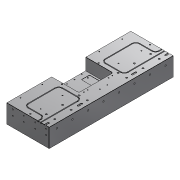
# Autodesk Inventor part: BC-10001
Saved by Autodesk Inventor 2016 (Build 200138000, 138)
## iProperties
Created: 2015-11-16
Part Number: BC-10001
Project: DIPOLO BC-3T- SIRIUS
Cost Center: 1504002005
Material: Aço Carbono AISI 1006
Document SubType Name: Modeling
Designer: reinaldo.basilio
Density: 7.872 g/cm^3
Appearance: Silver
Mass: 270714 g
Surface Area: 10813.1 cm^2
Volume: 34389.5 cm^3
Description: Base de referência de montagem do BC.
RuleStatus: InUse
AfterMaterialChange0: file://_iMaterial
AfterAnyiPropertyChange0: file://_iMaterial
AfterDocNew0: file://_Naming_par
AfterDocNew1: file://_NameStart
AfterDocNew2: file://_NameStart1
AfterDocNew3: file://_Materiais
DocNumber: XXXXX-XXX-XXXX-00-001.ipt
Folder: .
Title: DIPOLO BC-3T- SIRIUS
Author: reinaldo.basilio
Subject: BC-10001
Autodesk Inventor part; units mm, degrees
ref_plane "YZ Plane" through (0, 0, 0) normal (1, 0, 0) x (0, 1, 0)
ref_plane "XZ Plane" through (0, 0, 0) normal (0, 1, 0) x (-1, 0, 0)
ref_plane "XY Plane" through (0, 0, 0) normal (0, 0, 1) x (1, 0, 0)
sketch "Sketch5" plane through (0, 0, 0) normal (0, 0, 1) x (1, 0, 0)
  line L0 (-456.5, 228) -> (456.5, 228)
  line L1 (456.5, 228) -> (456.5, -55)
  line L2 (456.5, -55) -> (-456.5, -55)
  line L3 (-456.5, -55) -> (-456.5, 228)
  point P0 (0, 0)
  point P1 (0, 228)
  dimension "d8" = 913
  dimension "d154" = 55
  dimension "d523" = 283
  constraints: 8 end point, 2 parallel, 1 horizontal, 1 midpoint, 1 perpendicular, 1 vertical alignment
  measures "d8" distance of L0.start L0.end
  measures "d154" distance from line of L2 point (0, 0)
  measures "d523" distance of L0.end L1.end
extrude "Extrusion5" add sketch "Sketch5" along normal blind 137.5
sketch "Sketch7" plane through (0, 0, 137.5) normal (0, 0, 1) x (1, 0, 0)
  line L0 (125, -55) -> (125, 115)
  line L1 (0, 0) -> (0, 57.6278)
  line L2 (-125, -55) -> (-125, 115)
  line L3 (125, 115) -> (-125, 115)
  line L4 (125, -55) -> (-125, -55)
  line L5 (-456.5, 228) -> (-456.5, -55)
  line L6 (456.5, 228) -> (-456.5, 228) projected
  line L7 (-456.5, -55) -> (456.5, -55) projected
  point P0 (0, 115)
  point P1 (0, 28.8139)
  point P2 (0, -55)
  point P3 (0, -55)
  point P4 (0, 228)
  point P5 (0, 228)
  dimension "d76" = 250
  dimension "d77" = 170
  constraints: 12 end point, 6 midpoint, 4 vertical alignment, 2 vertical, 1 collinear, 1 horizontal, 1 symmetric about line
  measures "d76" distance of L0.end L2.end
  measures "d77" distance of L0.start L0.end
extrude "Extrusion7" cut sketch "Sketch7" against normal blind 87.5
sketch "Sketch11" plane through (0, 0, 50) normal (0, 0, 1) x (1, 0, 0)
  line L0 (90, 145) -> (-105, 145)
  line L1 (52.5, -55) -> (-52.5, -55) construction
  line L2 (-52.5, -55) -> (-52.5, 55)
  line L3 (-52.5, 55) -> (52.5, 55) construction
  line L4 (52.5, 55) -> (52.5, -55)
  line L5 (112.5, -45) -> (52.5, -45)
  line L6 (52.5, -45) -> (52.5, 45)
  line L7 (52.5, 45) -> (112.5, 45)
  line L8 (112.5, 45) -> (112.5, -45)
  line L9 (-125, -55) -> (-125, 115)
  line L10 (125, 115) -> (125, -55) projected
  line L11 (-125, -55) -> (-125, 115) projected
  line L12 (-125, 115) -> (125, 115) projected
  line L13 (0, 55) -> (0, -3.7877) construction
  line L14 (-112.5, -45) -> (-52.5, -45)
  line L15 (-52.5, 45) -> (-112.5, 45)
  line L16 (-112.5, 45) -> (-112.5, -45)
  line L17 (-52.5, -45) -> (-52.5, 45)
  line L18 (125, -55) -> (-125, -55) projected
  circle A0 centre (112.5, -45) radius 4
  circle A1 centre (52.5, -45) radius 4
  circle A2 centre (52.5, 45) radius 4
  circle A3 centre (112.5, 45) radius 4
  point P0 (112.5, 0)
  point P1 (52.5, 0)
  point P2 (0, 115)
  dimension "d55" = 110
  dimension "d56" = 105
  dimension "d58" = 60
  dimension "d59" = 90
  dimension "d156" = 72.5
  dimension "d158" = 72.5
  dimension "d160" = 60
  dimension "d225" = 55
  dimension "d310" = 8
  constraints: 30 end point, 5 midpoint, 4 centre point, 4 coincident, 4 symmetric about line, 3 equal radius, 3 parallel, 2 horizontal, 2 horizontal alignment, 2 perpendicular, 1 collinear, 1 vertical, 1 vertical alignment
  measures "d55" distance of L3.end L1.start
  measures "d56" distance of L2.end L3.end
  measures "d58" distance of L6.end L7.end
  measures "d59" distance of L7.end L5.start
  measures "d156" distance between parallel lines of L10 L4
  measures "d158" distance between parallel lines of L11 L2
  measures "d160" distance of L15.start L16.start
  measures "d225" distance from line of point (52.5, 0) L18
  measures "d310" diameter of A0
extrude "Extrusion9" cut sketch "Sketch11" against normal blind 2 contours L14 L16 L15 L2 | L4 A1 L5 | L4 A2 L7 A3 L8 A0 L5 A1 | L4 L7 A2 | A0 L8 L5 | L7 L8 A3 picked at (54.7437, -43.5902) picked at (54.3738, 43.1262) picked at (109.8668, -44.7033) picked at (110.2563, 43.5902)
fillet "Fillet2" radius 4 8 edges at (112.5, 45, 49) (52.5, 45, 49) (-112.5, 45, 49) (-52.5, 45, 49) (-112.5, -45, 49) (52.5, -45, 49) (-52.5, -45, 49) (112.5, -45, 49)
sketch "Sketch12" plane through (0, 0, 50) normal (0, 0, 1) x (1, 0, 0)
  line L0 (-434.5, -55) -> (478.5, -55)
  circle A0 centre (90.5, -35) radius 4.25
  circle A1 centre (90.5, 35) radius 4.25
  circle A2 centre (-90.5, -35) radius 4
  circle A3 centre (-90.5, 35) radius 4
  line L1 (-52.5, 41) -> (-52.5, -41)
  line L2 (52.5, -41) -> (52.5, 41)
  line L3 (125, -55) -> (-125, -55)
  line L4 (52.5, 0) -> (-52.5, 0) construction
  point P0 (0, -55)
  point P1 (0, 0)
  dimension "d64" = 70
  dimension "d65" = 90.5
  dimension "d66" = 8.5
  dimension "d157" = 90.5
  dimension "d270" = 55
  dimension "d271" = 35
  constraints: 10 end point, 4 centre point, 4 midpoint, 3 vertical alignment, 2 horizontal alignment, 1 equal radius, 3 other
  measures "d64" distance of A0.centre A1.centre
  measures "d65" horizontal distance of point (0, 0) A0.centre
  measures "d66" diameter of A0
  measures "d157" horizontal distance of point (0, 0) A3.centre
  measures "d270" distance from line of point (0, 0) L0
  measures "d271" vertical distance of point (0, 0) A0.centre
hole "Hole2" at (90.5, -35, 50) at (90.5, 35, 50) at (-90.5, 35, 50) at (-90.5, -35, 50) direction (0, 0, -1) diameter 8.376 depth 30 tip angle 118 thread size "M10x1.5" class "6H" standard "ISO Metric profile"
fillet "Fillet4" radius 10 2 edges at (125, 115, 93.75) (-125, 115, 93.75)
sketch "Sketch16" plane through (0, 0, 137.5) normal (0, 0, 1) x (1, 0, 0)
  line L0 (125, 105) -> (125, -55) projected
  line L1 (-456.5, -55) -> (-125, -55) projected
  circle A0 centre (0, 0) radius 8.7018
  line L2 (456.2612, -43.3901) -> (126.3743, -52.0283)
  line L3 (126.3743, -52.0283) -> (123.6257, 52.9357)
  line L4 (123.6257, 52.9357) -> (453.5127, 61.5739)
  line L5 (453.5127, 61.5739) -> (456.2612, -43.3901)
  circle A1 centre (440, 72.475) radius 5
  circle A2 centre (440, 72.475) radius 11.251
  line L6 (125, 0.4537) -> (454.8869, 9.0919)
  circle A3 centre (134.9966, 0.7155) radius 5
  line L7 (0, 0) -> (0, -90.9039)
  arc A4 (0, 0) -> (607.3073, 10.7125) centre (0, 17220) ccw construction
  line L8 (0, 0) -> (517.2786, 0) construction
  circle A5 centre (-440, 72.475) radius 11.251
  circle A6 centre (-134.9966, 0.7155) radius 5
  circle A7 centre (-440, 72.475) radius 11.251
  circle A8 centre (-134.9966, 0.7155) radius 5
  line L9 (125, 0.4537) -> (124.2986, 0.4537)
  line L10 (456.5, -55) -> (456.5, 228) projected
  point P0 (0, 0)
  point P1 (-456.5, 228)
  dimension "d95" = 55
  dimension "d100" = 10
  dimension "d117" = 105
  dimension "d119" = 17220
  dimension "d123" = 1.5
  dimension "d144" = 10
  dimension "d147" = 52.5
  dimension "d151" = 283
  dimension "d152" = 330
  dimension "d198" = 16.5
  dimension "d199" = 72.475
  dimension "d200" = 22.5021
  dimension "d201" = 134.9966
  dimension "d202" = 440
  constraints: 16 end point, 9 centre point, 4 parallel, 3 midpoint, 3 point on circle, 3 symmetric about line, 2 coincident, 2 concentric, 2 point on line, 1 horizontal, 1 perpendicular, 1 tangent, 1 vertical, 1 vertical alignment, 3 other
  measures "d95" distance from line of L7.start L1
  measures "d100" diameter of A1
  measures "d117" distance between parallel lines of L4 L2
  measures "d119" radius of A4
  measures "d123" angle of L6 L8
  measures "d144" diameter of A3
  measures "d147" distance between parallel lines of L4 L6
  measures "d151" distance of point (-456.5, 228) L1.start
  measures "d152" distance between parallel lines of L3 L5
  measures "d198" distance from line of L10 A1.centre
  measures "d199" vertical distance of A2.centre L7.start
  measures "d200" diameter of A2
  measures "d201" horizontal distance of L7.start A3.centre
  measures "d202" horizontal distance of L7.start A1.centre
hole "Hole3_ref angular" at (440, 72.475, 137.5) at (-440, 72.475, 137.5) at (134.9966, 0.7155, 137.5) at (-134.9966, 0.7155, 137.5) direction (0, 0, -1) diameter 10 depth 10
sketch "Sketch17" plane through (-456.5, -55, 0) normal (0, -1, 0) x (1, 0, 0)
  line L0 (581.5, 137.5) -> (581.5, 50)
  line L1 (581.5, 50) -> (331.5, 50)
  line L2 (331.5, 50) -> (331.5, 137.5)
  line L3 (0, 137.5) -> (331.5, 137.5)
  line L4 (0, 0) -> (0, 137.5)
  line L5 (913, 0) -> (0, 0)
  line L6 (913, 0) -> (913, 137.5)
  line L7 (581.5, 137.5) -> (913, 137.5)
  point P0 (456.5, 0)
  constraints: 16 end point
extrude "Extrusion11" add sketch "Sketch17" along normal blind 30
sketch "Sketch10" plane through (-456.5, -85, 0) normal (0, -1, 0) x (1, 0, 0)
  circle A0 centre (406.5, 25) radius 5
  circle A1 centre (506.5, 25) radius 5
  line L0 (913, 0) -> (0, 0)
  line L1 (581.5, 50) -> (331.5, 50)
  line L2 (581.5, 137.5) -> (581.5, 50) projected
  line L3 (581.5, 50) -> (331.5, 50) projected
  line L4 (331.5, 50) -> (331.5, 137.5) projected
  line L5 (331.5, 137.5) -> (0, 137.5) projected
  line L6 (0, 137.5) -> (0, 0) projected
  line L7 (0, 0) -> (913, 0) projected
  line L8 (913, 0) -> (913, 137.5) projected
  line L9 (913, 137.5) -> (581.5, 137.5) projected
  point P0 (456.5, 0)
  dimension "d44" = 10
  dimension "d319" = 50
  dimension "d320" = 100
  dimension "d321" = 50
  dimension "d322" = 25
  constraints: 4 end point, 2 centre point, 1 equal radius, 1 horizontal alignment
  measures "d44" diameter of A0
  measures "d319" distance between parallel lines of L0 L1
  measures "d320" distance of A1.centre A0.centre
  measures "d321" horizontal distance of A0.centre point (456.5, 0)
  measures "d322" distance from line of L0 A0.centre
hole "Hole1" at (-50, -85, 25) at (50, -85, 25) direction (0, 1, 0) diameter 8.376 depth 30 tip angle 118 thread size "M10x1.5" class "6H" standard "ANSI Metric M Profile"
sketch "Sketch18" plane through (0, 0, 137.5) normal (0, 0, 1) x (1, 0, 0)
  line L0 (135.1275, -4.2828) -> (125.282, -10.3161)
  line L1 (125.282, -10.3161) -> (126.4266, -54.0276)
  line L2 (157.2017, -83.232) -> (126.4266, -54.0276)
  line L3 (157.2017, -83.232) -> (427.1091, -76.1643)
  line L4 (456.3136, -45.3892) -> (427.1091, -76.1643)
  line L5 (456.3136, -45.3892) -> (453.4603, 63.5734)
  line L6 (422.6852, 92.7778) -> (453.4603, 63.5734)
  line L7 (422.6852, 92.7778) -> (152.7778, 85.71)
  line L8 (123.5734, 54.935) -> (152.7778, 85.71)
  line L9 (123.5734, 54.935) -> (124.718, 11.2235)
  line L10 (124.718, 11.2235) -> (134.8657, 5.7137)
  arc A0 (135.1275, -4.2828) -> (134.8657, 5.7137) centre (134.9966, 0.7155) ccw
  circle A1 centre (370.5174, 79.4076) radius 4
  line L11 (289.9435, 4.7729) -> (269.2931, 4.2321)
  circle A2 centre (374.313, -65.5427) radius 4
  line L12 (289.9435, 4.7729) -> (290.4494, -14.5478)
  circle A3 centre (205.5739, 75.0884) radius 4
  circle A4 centre (209.3696, -69.8619) radius 4
  arc A5 (365.3739, 75.2716) -> (375.8703, 75.5464) centre (370.6221, 75.409) ccw
  line L13 (365.3739, 75.2716) -> (365.1645, 83.2688)
  arc A6 (375.6609, 83.5437) -> (365.1645, 83.2688) centre (370.4127, 83.4063) ccw
  line L14 (375.6609, 83.5437) -> (375.8703, 75.5464)
  arc A7 (379.4565, -61.4066) -> (368.9601, -61.6815) centre (374.2083, -61.544) ccw
  line L15 (379.6659, -69.4039) -> (379.4565, -61.4066)
  arc A8 (369.1695, -69.6787) -> (379.6659, -69.4039) centre (374.4177, -69.5413) ccw
  line L16 (368.9601, -61.6815) -> (369.1695, -69.6787)
  line L17 (204.2261, -73.9979) -> (204.0166, -66.0007)
  arc A9 (214.5131, -65.7258) -> (204.0166, -66.0007) centre (209.2649, -65.8632) ccw
  line L18 (214.5131, -65.7258) -> (214.7225, -73.7231)
  arc A10 (204.2261, -73.9979) -> (214.7225, -73.7231) centre (209.4743, -73.8605) ccw
  arc A11 (200.4304, 70.9524) -> (210.9268, 71.2272) centre (205.6786, 71.0898) ccw
  line L19 (200.221, 78.9496) -> (200.4304, 70.9524)
  line L20 (210.9268, 71.2272) -> (210.7174, 79.2245)
  arc A12 (210.7174, 79.2245) -> (200.221, 78.9496) centre (205.4692, 79.0871) ccw
  line L21 (0, 0) -> (0, -229.0082) construction
  line L22 (-123.5734, 54.935) -> (-124.718, 11.2235)
  line L23 (-124.718, 11.2235) -> (-134.8657, 5.7137)
  arc A13 (-134.8657, 5.7137) -> (-135.1275, -4.2828) centre (-134.9966, 0.7155) ccw
  line L24 (-123.5734, 54.935) -> (-152.7778, 85.71)
  line L25 (-422.6852, 92.7778) -> (-152.7778, 85.71)
  line L26 (-157.2017, -83.232) -> (-427.1091, -76.1643)
  circle A14 centre (-209.3696, -69.8619) radius 4
  circle A15 centre (-205.5739, 75.0884) radius 4
  line L27 (-456.3136, -45.3892) -> (-427.1091, -76.1643)
  line L28 (-456.3136, -45.3892) -> (-453.4603, 63.5734)
  line L29 (-422.6852, 92.7778) -> (-453.4603, 63.5734)
  circle A16 centre (-370.5174, 79.4076) radius 4
  circle A17 centre (-374.313, -65.5427) radius 4
  line L30 (-135.1275, -4.2828) -> (-125.282, -10.3161)
  line L31 (-125.282, -10.3161) -> (-126.4266, -54.0276)
  line L32 (-157.2017, -83.232) -> (-126.4266, -54.0276)
  line L33 (-108.5, 45) -> (-56.5, 45) projected
  dimension "d177" = 8
  dimension "d178" = 10.5
  dimension "d179" = 10.5
  dimension "d180" = 10.5
  dimension "d181" = 10.5
  dimension "d182" = 8
  dimension "d183" = 8
  dimension "d188" = 84.3696
  dimension "d189" = 80.5739
  dimension "d190" = 145
  dimension "d520" = 82.5
  dimension "d521" = 82.5
  constraints: 66 end point, 21 symmetric about line, 20 point on circle, 18 centre point, 1 vertical, 9 other
  measures "d177" diameter of A1
  measures "d178" distance between parallel lines of L13 L14
  measures "d179" distance between parallel lines of L16 L15
  measures "d180" distance between parallel lines of L18 L17
  measures "d181" distance between parallel lines of L20 L19
  measures "d182" distance of L14.start L14.end
  measures "d183" distance of L13.start L13.end
  measures "d188" horizontal distance of L12.start A2.centre
  measures "d189" horizontal distance of A4.centre L12.start
  measures "d190" distance of A2.centre A1.centre
  measures "d520" distance from line of L12 A4.centre
  measures "d521" distance from line of L12 A2.centre
hole "Hole5" at (209.3696, -69.8619, 137.5) at (374.313, -65.5427, 137.5) at (370.5174, 79.4076, 137.5) at (205.5739, 75.0884, 137.5) at (-374.313, -65.5427, 137.5) at (-370.5174, 79.4076, 137.5) at (-205.5739, 75.0884, 137.5) at (-209.3696, -69.8619, 137.5) direction (0, 0, -1) diameter 6.647 depth 25 tip angle 118 thread size "M8x1.25" class "6H" standard "ANSI Metric M Profile"
sketch "Sketch19" plane through (0, 0, 137.5) normal (0, 0, 1) x (1, 0, 0)
  line L0 (-115, 115) -> (115, 115) projected
  circle A0 centre (27.5, 171.5) radius 4
  circle A1 centre (-27.5, 171.5) radius 4
  line L1 (456.5, 228) -> (-456.5, 228) projected
  point P0 (0, 0)
  dimension "d203" = 8
  dimension "d205" = 27.5
  dimension "d206" = 56.5
  dimension "d306" = 113
  dimension "d307" = 55
  constraints: 2 centre point, 1 equal radius, 1 horizontal alignment
  measures "d203" diameter of A0
  measures "d205" horizontal distance of A1.centre point (0, 0)
  measures "d206" distance from line of L0 A1.centre
  measures "d306" distance between parallel lines of L1 L0
  measures "d307" distance of A1.centre A0.centre
hole "Hole6" at (27.5, 171.5, 137.5) at (-27.5, 171.5, 137.5) direction (0, 0, -1) diameter 6.647 depth 25 tip angle 118 thread size "M8x1.25" class "6H" standard "ANSI Metric M Profile"
sketch "Sketch20" plane through (0, 0, 137.5) normal (0, 0, 1) x (1, 0, 0)
  line L0 (125, 105) -> (125, -85) projected
  line L1 (456.5, 228) -> (456.5, -85) projected
  line L2 (456.5, 228) -> (-456.5, 228) projected
  line L3 (-115, 115) -> (115, 115) projected
  arc A0 (155, 26.75) -> (185, -3.25) centre (185, 26.75) ccw
  line L4 (185, -3.25) -> (381.5, -3.25)
  line L5 (185, 168.75) -> (456.5, 168.75)
  line L6 (381.5, 3.25) -> (185, 3.25)
  arc A1 (161.5, 26.75) -> (185, 3.25) centre (185, 26.75) ccw
  line L7 (185, 162.25) -> (456.5, 162.25)
  line L8 (0, 115) -> (0, 228)
  line L9 (456.5, 162.25) -> (456.5, 168.75)
  circle A2 centre (0, 0) radius 9.0257
  line L10 (125, -85) -> (-125, -85) projected
  line L11 (0, 0) -> (0, -43.6286) construction
  arc A3 (185, 168.75) -> (155, 138.75) centre (185, 138.75) ccw
  arc A4 (185, 162.25) -> (161.5, 138.75) centre (185, 138.75) ccw
  line L12 (161.5, 26.75) -> (161.5, 138.75)
  line L13 (155, 26.75) -> (155, 138.75)
  line L14 (405, 26.75) -> (405, 118.75)
  line L15 (411.5, 26.75) -> (411.5, 118.75)
  arc A5 (381.5, -3.25) -> (411.5, 26.75) centre (381.5, 26.75) ccw
  arc A6 (381.5, 3.25) -> (405, 26.75) centre (381.5, 26.75) ccw
  line L16 (435, 142.25) -> (456.5, 142.25)
  line L17 (435, 148.75) -> (456.5, 148.75)
  arc A7 (435, 142.25) -> (411.5, 118.75) centre (435, 118.75) ccw
  arc A8 (435, 148.75) -> (405, 118.75) centre (435, 118.75) ccw
  line L18 (456.5, -85) -> (125, -85) projected
  line L19 (456.5, 142.25) -> (456.5, 148.75)
  line L20 (456.5, 165.5) -> (451.5764, 165.5) construction
  line L21 (456.5, 145.5) -> (447.5617, 145.5) construction
  arc A9 (-185, -3.25) -> (-155, 26.75) centre (-185, 26.75) ccw
  line L22 (-185, -3.25) -> (-381.5, -3.25)
  line L23 (-185, 168.75) -> (-456.5, 168.75)
  line L24 (-381.5, 3.25) -> (-185, 3.25)
  arc A10 (-185, 3.25) -> (-161.5, 26.75) centre (-185, 26.75) ccw
  line L25 (-185, 162.25) -> (-456.5, 162.25)
  line L26 (-456.5, 162.25) -> (-456.5, 168.75)
  arc A11 (-155, 138.75) -> (-185, 168.75) centre (-185, 138.75) ccw
  arc A12 (-161.5, 138.75) -> (-185, 162.25) centre (-185, 138.75) ccw
  line L27 (-161.5, 26.75) -> (-161.5, 138.75)
  line L28 (-155, 26.75) -> (-155, 138.75)
  line L29 (-405, 26.75) -> (-405, 118.75)
  line L30 (-411.5, 26.75) -> (-411.5, 118.75)
  arc A13 (-411.5, 26.75) -> (-381.5, -3.25) centre (-381.5, 26.75) ccw
  arc A14 (-405, 26.75) -> (-381.5, 3.25) centre (-381.5, 26.75) ccw
  line L31 (-435, 142.25) -> (-456.5, 142.25)
  line L32 (-435, 148.75) -> (-456.5, 148.75)
  arc A15 (-411.5, 118.75) -> (-435, 142.25) centre (-435, 118.75) ccw
  arc A16 (-405, 118.75) -> (-435, 148.75) centre (-435, 118.75) ccw
  line L33 (-456.5, 142.25) -> (-456.5, 148.75)
  point P0 (0, 0)
  point P1 (0, 171.5)
  dimension "d217" = 6.5
  dimension "d224" = 85
  dimension "d442" = 6.5
  dimension "d443" = 30
  dimension "d444" = 45
  dimension "d446" = 23.5
  dimension "d448" = 6.5
  dimension "d449" = 23.5
  dimension "d450" = 30
  dimension "d451" = 301.5
  dimension "d452" = 30
  dimension "d453" = 30
  dimension "d456" = 59.25
  dimension "d457" = 30
  dimension "d458" = 23.5
  dimension "d459" = 23.5
  dimension "d505" = 81.75
  dimension "d506" = 6.5
  dimension "d507" = 6.5
  dimension "d509" = 62.5
  dimension "d510" = 20
  dimension "d511" = 159
  constraints: 56 end point, 32 point on circle, 26 symmetric about line, 17 centre point, 12 tangent, 5 horizontal, 5 midpoint, 3 parallel, 3 perpendicular, 2 point on line, 1 coincident, 1 collinear, 1 vertical, 8 other
  measures "d217" distance between parallel lines of L6 L4
  measures "d224" distance from line of L11.start L10
  measures "d442" distance between parallel lines of L15 L14
  measures "d443" radius of A5
  measures "d444" distance between parallel lines of L1 L15
  measures "d446" radius of A6
  measures "d448" distance between parallel lines of L17 L16
  measures "d449" radius of A7
  measures "d450" radius of A8
  measures "d451" distance between parallel lines of L13 L1
  measures "d452" distance between parallel lines of L13 L0
  measures "d453" radius of A0
  measures "d456" distance between parallel lines of L2 L5
  measures "d457" radius of A3
  measures "d458" radius of A4
  measures "d459" radius of A1
  measures "d505" distance between parallel lines of L4 L18
  measures "d506" distance between parallel lines of L7 L5
  measures "d507" distance between parallel lines of L13 L12
  measures "d509" distance between parallel lines of L2 L20
  measures "d510" distance between parallel lines of L20 L21
  measures "d511" distance between parallel lines of L7 L6
extrude "Extrusion12_Est. Térmica" cut sketch "Sketch20" against normal blind 6.5 contours L1 L7 A4 L12 A1 L6 A6 L14 A8 L17 L16 A7 L15 A5 L4 A0 L13 A3 L5 | A2 | L22 A13 L30 A15 L31 L33 L32 A16 L29 A14 L24 A10 L27 A12 L25 L26 L23 A11 L28 A9
sketch "Sketch21" plane through (456.5, 228, 137.5) normal (1, 0, 0) x (0, 0, -1)
  line L0 (0, 0) -> (0, -313)
  line L1 (137.5, -313) -> (0, -313)
  circle A0 centre (20, -268) radius 4
  circle A1 centre (20, -188) radius 4
  circle A2 centre (60, -268) radius 4
  circle A3 centre (60, -188) radius 4
  line L2 (-9.7116, -228) -> (31.8893, -228)
  line L3 (137.5, 0) -> (0, 0) projected
  circle A4 centre (20, -102.5) radius 4
  circle A5 centre (20, -22.5) radius 4
  circle A6 centre (60, -102.5) radius 4
  circle A7 centre (60, -22.5) radius 4
  line L4 (-9.7116, -62.5) -> (31.8893, -62.5)
  point P0 (137.5, -156.5)
  dimension "d221" = 80
  dimension "d222" = 85
  dimension "d223" = 313
  dimension "d226" = 40
  dimension "d228" = 40
  dimension "d230" = 8
  dimension "d324" = 20
  dimension "d513" = 80
  dimension "d514" = 40
  dimension "d515" = 40
  dimension "d516" = 40
  dimension "d517" = 8
  dimension "d518" = 62.5
  constraints: 8 centre point, 8 end point, 6 equal radius, 5 vertical alignment, 4 horizontal alignment, 2 horizontal
  measures "d221" distance of A2.centre A3.centre
  measures "d222" distance between parallel lines of L2 L1
  measures "d223" distance of L3.start L1.start
  measures "d226" distance from line of A0.centre L2
  measures "d228" distance of A2.centre A0.centre
  measures "d230" diameter of A1
  measures "d324" distance from line of L0 A0.centre
  measures "d513" distance of A6.centre A7.centre
  measures "d514" distance from line of A4.centre L4
  measures "d515" distance from line of A5.centre L4
  measures "d516" distance of A6.centre A4.centre
  measures "d517" diameter of A5
  measures "d518" distance between parallel lines of L3 L4
hole "Hole7" at (456.5, -40, 117.5) at (456.5, -40, 77.5) at (456.5, 40, 77.5) at (456.5, 40, 117.5) at (456.5, 125.5, 117.5) at (456.5, 205.5, 117.5) at (456.5, 205.5, 77.5) at (456.5, 125.5, 77.5) direction (-1, 0, 0) diameter 8.376 depth 20 tip angle 118 thread size "M10x1.5" class "6H" standard "ANSI Metric M Profile"
sketch "Sketch22" plane through (-456.5, 228, 0) normal (-1, 0, 0) x (0, 0, 1)
  circle A0 centre (117.5, -188) radius 4.188
  circle A1 centre (117.5, -268) radius 4.188
  circle A2 centre (77.5, -268) radius 4.188
  circle A3 centre (77.5, -188) radius 4.188
  circle A4 centre (117.5, -188) radius 4.188 projected
  circle A5 centre (117.5, -268) radius 4.188 projected
  circle A6 centre (77.5, -268) radius 4.188 projected
  circle A7 centre (77.5, -188) radius 4.188 projected
  circle A8 centre (117.5, -22.5) radius 5
  circle A9 centre (77.5, -22.5) radius 5
  circle A10 centre (117.5, -102.5) radius 5
  circle A11 centre (77.5, -102.5) radius 5
  circle A12 centre (117.5, -22.5) radius 4.188 projected
  circle A13 centre (117.5, -102.5) radius 4.188 projected
  circle A14 centre (77.5, -102.5) radius 4.188 projected
  circle A15 centre (77.5, -22.5) radius 4.188 projected
  point P0 (0, -228)
  dimension "d519" = 10
  constraints: 8 centre point, 8 concentric, 7 equal radius
  measures "d519" diameter of A8
hole "Hole8" at (-456.5, -40, 117.5) at (-456.5, 40, 117.5) at (-456.5, 40, 77.5) at (-456.5, -40, 77.5) at (-456.5, 125.5, 117.5) at (-456.5, 125.5, 77.5) at (-456.5, 205.5, 77.5) at (-456.5, 205.5, 117.5) direction (1, 0, 0) diameter 8.376 depth 20 tip angle 118 thread size "M10x1.5" class "6H" standard "ANSI Metric M Profile"
sketch "Sketch23" plane through (0, 0, 0) normal (0, 0, -1) x (-1, 0, 0)
  line L0 (456.5, 228) -> (-456.5, 228) projected
  line L1 (-456.5, 228) -> (-456.5, -85) projected
  circle A0 centre (-384, 196.75) radius 7.5
  circle A1 centre (-384, 134.25) radius 7.5
  circle A2 centre (-264, 196.75) radius 7.5
  circle A3 centre (-264, 134.25) radius 7.5
  circle A4 centre (-144, 196.75) radius 7.5
  circle A5 centre (-144, 134.25) radius 7.5
  circle A6 centre (-144, 196.75) radius 7.5
  circle A7 centre (-144, 134.25) radius 7.5
  circle A8 centre (-264, 134.25) radius 7.5
  circle A9 centre (-264, 196.75) radius 7.5
  circle A10 centre (-384, 196.75) radius 7.5
  circle A11 centre (-384, 134.25) radius 7.5
  circle A12 centre (384, 196.75) radius 7.5
  circle A13 centre (384, 134.25) radius 7.5
  circle A14 centre (264, 196.75) radius 7.5
  circle A15 centre (264, 134.25) radius 7.5
  circle A16 centre (144, 196.75) radius 7.5
  circle A17 centre (144, 134.25) radius 7.5
  circle A18 centre (144, 196.75) radius 7.5
  circle A19 centre (144, 134.25) radius 7.5
  circle A20 centre (264, 134.25) radius 7.5
  circle A21 centre (264, 196.75) radius 7.5
  circle A22 centre (384, 196.75) radius 7.5
  circle A23 centre (384, 134.25) radius 7.5
  line L2 (456.5, -85) -> (456.5, 228) projected
  line L3 (0, 228) -> (0, 265.8174) construction
  dimension "d246" = 120
  dimension "d247" = 120
  dimension "d248" = 31.25
  dimension "d257" = 62.5
  dimension "d258" = 15
  dimension "d390" = 120
  dimension "d391" = 120
  dimension "d395" = 192.5
  dimension "d396" = 72.5
  dimension "d397" = 192.5
  constraints: 24 centre point, 11 concentric, 11 equal radius, 10 horizontal alignment, 7 vertical alignment, 2 end point, 1 midpoint, 1 vertical
  measures "d246" distance of A5.centre A3.centre
  measures "d247" distance of A3.centre A1.centre
  measures "d248" distance from line of A0.centre L0
  measures "d257" distance of A1.centre A0.centre
  measures "d258" diameter of A0
  measures "d390" distance of A17.centre A15.centre
  measures "d391" distance of A23.centre A15.centre
  measures "d395" distance from line of A9.centre L1
  measures "d396" distance from line of L1 A0.centre
  measures "d397" distance from line of L2 A14.centre
hole "Hole9" at (384, 196.75, 0) at (384, 134.25, 0) at (264, 134.25, 0) at (264, 196.75, 0) at (144, 134.25, 0) at (144, 196.75, 0) at (-144, 134.25, 0) at (-144, 196.75, 0) at (-264, 134.25, 0) at (-264, 196.75, 0) at (-384, 134.25, 0) at (-384, 196.75, 0) direction (0, 0, 1) diameter 12.5 end through all counterbore diameter 20 counterbore depth 60 clearance for "Socket Head Cap Screw DIN EN ISO 4762" size "M12" standard "DIN"
sketch "Sketch24" plane through (0, 0, 50) normal (0, 0, 1) x (1, 0, 0)
  line L0 (-115, 115) -> (115, 115) projected
  circle A0 centre (-27.5, 70) radius 4
  circle A1 centre (27.5, 70) radius 4
  line L1 (-52.5, 115) -> (52.5, 115)
  line L2 (52.5, 115) -> (52.5, 55)
  line L3 (52.5, 55) -> (-52.5, 55)
  line L4 (-52.5, 55) -> (-52.5, 115)
  line L5 (-115, 115) -> (115, 115) projected
  line L6 (125, -85) -> (-125, -85) projected
  circle A2 centre (-27.5, -70) radius 4
  circle A3 centre (27.5, -70) radius 4
  circle A4 centre (-90, -79) radius 4
  circle A5 centre (90, -79) radius 4
  point P0 (0, 0)
  point P1 (0, 115)
  point P2 (0, 115)
  dimension "d272" = 105
  dimension "d273" = 60
  dimension "d274" = 55
  dimension "d275" = 27.5
  dimension "d276" = 8
  dimension "d277" = 45
  dimension "d289" = 8
  dimension "d290" = 15
  dimension "d325" = 6
  dimension "d326" = 90
  dimension "d327" = 180
  constraints: 8 end point, 6 centre point, 4 equal radius, 3 horizontal alignment, 2 midpoint, 2 parallel, 2 vertical alignment, 1 coincident, 1 collinear, 1 horizontal, 1 perpendicular
  measures "d272" distance of L2.end L3.end
  measures "d273" distance of L3.end L1.start
  measures "d274" distance of A1.centre A0.centre
  measures "d275" horizontal distance of point (0, 0) A0.centre
  measures "d276" diameter of A0
  measures "d277" distance from line of A0.centre L0
  measures "d289" diameter of A2
  measures "d290" distance from line of A3.centre L6
  measures "d325" distance from line of A4.centre L6
  measures "d326" horizontal distance of point (0, 0) A4.centre
  measures "d327" distance of A5.centre A4.centre
hole "Hole10" at (-27.5, 70, 50) at (27.5, 70, 50) at (27.5, -70, 50) at (-27.5, -70, 50) at (-90, -79, 50) at (90, -79, 50) direction (0, 0, -1) diameter 6.647 depth 15 tip angle 118 thread size "M8x1.25" class "6H" standard "ISO Metric profile"
chamfer "Chamfer3" distance 1 angle 45 5 edges at (-125, 10, 137.5) (-122.0711, 112.0711, 137.5) (0, 115, 137.5) (122.0711, 112.0711, 137.5) (125, 10, 137.5)
sketch "Sketch25" plane through (0, 0, 137.5) normal (0, 0, 1) x (1, 0, 0)
  line L0 (115, 116) -> (-115, 116) projected
  line L1 (0, 0) -> (0, 181.9639)
  line L2 (-52.5, 0) -> (-52.5, 181.9639)
  line L3 (-67.5, 0) -> (-67.5, 181.9639)
  line L4 (-112.5, 0) -> (-112.5, 181.9639)
  circle A0 centre (-76.5, 131) radius 4
  circle A1 centre (-104.5, 131) radius 4
  circle A2 centre (76.5, 131) radius 4
  circle A3 centre (104.5, 131) radius 4
  line L5 (-68.5, 0) -> (-68.5, 181.9639)
  dimension "d291" = 52.5
  dimension "d292" = 15
  dimension "d293" = 60
  dimension "d294" = 45
  dimension "d295" = 28
  dimension "d297" = 8
  dimension "d298" = 15
  dimension "d308" = 1
  dimension "d309" = 8
  constraints: 10 end point, 4 centre point, 4 parallel, 2 symmetric about line, 1 equal radius, 1 horizontal alignment, 1 vertical, 2 other
  measures "d291" distance between parallel lines of L2 L1
  measures "d292" distance between parallel lines of L3 L2
  measures "d293" distance between parallel lines of L4 L2
  measures "d294" distance between parallel lines of L4 L3
  measures "d295" distance of A1.centre A0.centre
  measures "d297" diameter of A0
  measures "d298" distance from line of A0.centre L0
  measures "d308" distance between parallel lines of L5 L3
  measures "d309" distance from line of A0.centre L5
hole "Hole11" at (-104.5, 131, 137.5) at (-76.5, 131, 137.5) at (76.5, 131, 137.5) at (104.5, 131, 137.5) direction (0, 0, -1) diameter 6.647 depth 25 tip angle 118 thread size "M8x1.25" class "6H" standard "ISO Metric profile"
sketch "Sketch26" plane through (0, 0, 137.5) normal (0, 0, 1) x (1, 0, 0)
  circle A0 centre (-144, 134.25) radius 6.25 projected
  line L0 (-186.5, 196.75) -> (-211.5, 196.75) construction
  line L1 (-186.5, 202.75) -> (-211.5, 202.75)
  line L2 (-211.5, 190.75) -> (-186.5, 190.75)
  arc A1 (-186.5, 190.75) -> (-186.5, 202.75) centre (-186.5, 196.75) ccw
  arc A2 (-211.5, 202.75) -> (-211.5, 190.75) centre (-211.5, 196.75) ccw
  line L3 (-431.5, 196.75) -> (-456.5, 196.75) construction
  line L4 (-431.5, 202.75) -> (-456.5, 202.75)
  line L5 (-456.5, 190.75) -> (-431.5, 190.75)
  arc A3 (-431.5, 190.75) -> (-431.5, 202.75) centre (-431.5, 196.75) ccw
  arc A4 (-456.5, 202.75) -> (-456.5, 190.75) centre (-456.5, 196.75) ccw
  line L6 (0, 0) -> (0, 125.3683) construction
  line L7 (186.5, 196.75) -> (211.5, 196.75) construction
  line L8 (186.5, 202.75) -> (211.5, 202.75)
  line L9 (211.5, 190.75) -> (186.5, 190.75)
  arc A5 (186.5, 202.75) -> (186.5, 190.75) centre (186.5, 196.75) ccw
  arc A6 (211.5, 190.75) -> (211.5, 202.75) centre (211.5, 196.75) ccw
  line L10 (431.5, 196.75) -> (456.5, 196.75) construction
  line L11 (431.5, 202.75) -> (456.5, 202.75)
  line L12 (456.5, 190.75) -> (431.5, 190.75)
  arc A7 (431.5, 202.75) -> (431.5, 190.75) centre (431.5, 196.75) ccw
  arc A8 (456.5, 190.75) -> (456.5, 202.75) centre (456.5, 196.75) ccw
  line L13 (-456.5, 228) -> (-456.5, -85) projected
  line L14 (-456.5, 228) -> (-456.5, -85) projected
  circle A9 centre (-384, 196.75) radius 6.25 projected
  point P0 (-199, 196.75)
  point P1 (-444, 196.75)
  point P2 (-199, 196.75)
  point P3 (-444, 196.75)
  point P4 (199, 196.75)
  point P5 (444, 196.75)
  point P6 (199, 196.75)
  point P7 (444, 196.75)
  point P8 (-456.5, -68.25)
  point P9 (-456.5, 103.25)
  dimension "d311" = 12
  dimension "d312" = 12
  dimension "d313" = 25
  dimension "d314" = 25
  dimension "d317" = 257.5
  dimension "d318" = 12.5
  dimension "d463" = 0
  constraints: 34 end point, 16 point on circle, 16 symmetric about line, 8 centre point, 8 tangent, 4 coincident, 2 horizontal alignment, 2 midpoint, 2 parallel, 1 vertical, 4 other
  measures "d311" distance between parallel lines of L2 L1
  measures "d312" distance between parallel lines of L4 L5
  measures "d313" distance of L0.start L0.end
  measures "d314" distance of L3.start L3.end
  measures "d317" distance from line of L14 point (-199, 196.75)
  measures "d318" distance from line of L13 point (-444, 196.75)
  measures "d463" vertical distance of A9.centre point (-444, 196.75)
extrude "Extrusion13" cut sketch "Sketch26" against normal blind 5 contours A1 L2 A2 L1 | A3 L5 L13 L4 | L13 A4 | L8 A6 L9 A5 | L11 A8 L12 A7
sketch "Sketch27" plane through (0, 0, 132.5) normal (0, 0, 1) x (1, 0, 0)
  arc A0 (431.5, 202.75) -> (431.5, 190.75) centre (431.5, 196.75) ccw projected
  circle A1 centre (444, 196.75) radius 2
  circle A2 centre (199, 196.75) radius 2
  line L0 (456.5, 190.75) -> (431.5, 190.75) projected
  line L1 (211.5, 190.75) -> (186.5, 190.75) projected
  line L2 (0, 0) -> (0, 29.1293) construction
  circle A3 centre (-444, 196.75) radius 2
  circle A4 centre (-199, 196.75) radius 2
  line L3 (431.5, 202.75) -> (456.5, 202.75) projected
  line L4 (-211.5, 202.75) -> (-186.5, 202.75) projected
  line L5 (186.5, 202.75) -> (211.5, 202.75) projected
  point P0 (199, 190.75)
  point P1 (444, 202.75)
  point P2 (-199, 202.75)
  point P3 (199, 202.75)
  dimension "d328" = 4
  constraints: 4 centre point, 4 midpoint, 4 vertical alignment, 2 end point, 2 horizontal alignment, 2 symmetric about line, 1 equal radius, 1 vertical, 2 other
  measures "d328" diameter of A1
hole "Hole12" at (444, 196.75, 132.5) at (199, 196.75, 132.5) at (-199, 196.75, 132.5) at (-444, 196.75, 132.5) direction (0, 0, -1) diameter 3.242 depth 12 tip angle 118 thread size "M4x0.7" class "6H" standard "ISO Metric profile"
sketch "Sketch28" plane through (-456.5, -85, 0) normal (0, -1, 0) x (1, 0, 0)
  line L0 (331.5, 50) -> (331.5, 136.5) projected
  line L1 (330.5, 137.5) -> (0, 137.5) projected
  line L2 (0, 137.5) -> (0, 0) projected
  circle A0 centre (42.25, 121) radius 4
  circle A1 centre (124.25, 121) radius 4
  circle A2 centre (206.25, 121) radius 4
  circle A3 centre (288.25, 121) radius 4
  line L3 (456.5, 0) -> (456.5, -39.2028) construction
  circle A4 centre (870.75, 121) radius 4
  circle A5 centre (788.75, 121) radius 4
  circle A6 centre (706.75, 121) radius 4
  circle A7 centre (624.75, 121) radius 4
  line L4 (165.25, 137.5) -> (165.25, 146.8704) construction
  line L5 (0, 0) -> (913, 0) projected
  dimension "d336" = 331.5
  dimension "d337" = 82
  dimension "d338" = 82
  dimension "d340" = 82
  dimension "d341" = 8
  dimension "d375" = 41
  dimension "d525" = 16.5
  dimension "d526" = 121
  constraints: 8 centre point, 4 end point, 4 symmetric about line, 3 equal radius, 3 horizontal alignment, 2 vertical, 1 midpoint, 4 other
  measures "d336" distance between parallel lines of L0 L2
  measures "d337" distance of A2.centre A1.centre
  measures "d338" distance of A3.centre A2.centre
  measures "d340" distance of A0.centre A1.centre
  measures "d341" diameter of A0
  measures "d375" distance from line of A2.centre L4
  measures "d525" distance from line of A0.centre L1
  measures "d526" distance from line of A0.centre L5
hole "Hole13" at (-414.25, -85, 121) at (-332.25, -85, 121) at (-250.25, -85, 121) at (-168.25, -85, 121) at (168.25, -85, 121) at (250.25, -85, 121) at (332.25, -85, 121) at (414.25, -85, 121) direction (0, 1, 0) diameter 6.647 depth 25 tip angle 118 thread size "M8x1.25" class "6H" standard "ISO Metric profile"
sketch "Sketch29" plane through (0, 0, 0) normal (0, 0, -1) x (-1, 0, 0)
  line L0 (125, 33.5) -> (125, -126.5)
  circle A0 centre (0, 0) radius 4
  line L1 (456.2612, -43.3901) -> (126.3743, -52.0283) construction
  line L2 (126.3743, -52.0283) -> (123.6257, 52.9357) construction
  line L3 (123.6257, 52.9357) -> (453.5127, 61.5739) construction
  line L4 (453.5127, 61.5739) -> (456.2612, -43.3901) construction
  circle A1 centre (440, 72.475) radius 5
  circle A2 centre (440, 72.475) radius 11.251
  line L5 (125, 0.4537) -> (454.8869, 9.0919)
  circle A3 centre (134.9966, 0.7155) radius 5
  line L6 (0, 0) -> (0, -90.9039) construction
  arc A4 (0, 0) -> (604.7976, 10.6241) centre (0, 17220) ccw construction
  line L7 (0, 0) -> (517.2786, 0) construction
  circle A5 centre (-440, 72.475) radius 11.251
  circle A6 centre (-134.9966, 0.7155) radius 5
  circle A7 centre (-440, 72.475) radius 11.251
  circle A8 centre (-134.9966, 0.7155) radius 5
  line L8 (125, 0.4537) -> (124.2986, 0.4537)
  line L9 (456.5, -126.5) -> (456.5, 156.5)
  circle A9 centre (430, 8.4402) radius 4
  circle A10 centre (0, 0) radius 1.2468
  circle A11 centre (-430, 8.4402) radius 4
  circle A12 centre (0, 210) radius 4
  line L10 (456.5, -85) -> (-456.5, -85) projected
  point P0 (0, 0)
  point P1 (0, 0)
  point P2 (-456.5, 156.5)
  dimension "d350" = 10
  dimension "d351" = 105
  dimension "d352" = 17220
  dimension "d353" = 1.5
  dimension "d354" = 10
  dimension "d355" = 52.5
  dimension "d357" = 330
  dimension "d358" = 16.5
  dimension "d359" = 72.475
  dimension "d360" = 22.5021
  dimension "d361" = 134.9966
  dimension "d362" = 440
  dimension "d363" = 430
  dimension "d364" = 8
  dimension "d365" = 8
  dimension "d367" = 210
  dimension "d524" = 85
  constraints: 20 end point, 13 centre point, 4 parallel, 4 symmetric about line, 3 coincident, 3 midpoint, 3 point on circle, 3 point on line, 2 equal radius, 2 vertical alignment, 1 concentric, 1 horizontal, 1 perpendicular, 1 tangent, 1 vertical, 4 other
  measures "d350" diameter of A1
  measures "d351" distance between parallel lines of L3 L1
  measures "d352" radius of A4
  measures "d353" angle of L5 L7
  measures "d354" diameter of A3
  measures "d355" distance between parallel lines of L3 L5
  measures "d357" distance between parallel lines of L2 L4
  measures "d358" distance from line of L9 A1.centre
  measures "d359" vertical distance of A2.centre L6.start
  measures "d360" diameter of A2
  measures "d361" horizontal distance of L6.start A3.centre
  measures "d362" horizontal distance of L6.start A1.centre
  measures "d363" horizontal distance of L6.start A9.centre
  measures "d364" diameter of A9
  measures "d365" diameter of A0
  measures "d367" distance of A12.centre L6.start
  measures "d524" distance from line of L10 L6.start
hole "Hole14" at (0, 0, 0) at (-430, 8.4402, 0) at (0, 0, 0) at (0, 210, 0) at (430, 8.4402, 0) direction (0, 0, 1) diameter 8 depth 15 tip angle 118
sketch "Sketch30" plane through (-456.5, 228, 0) normal (0, 1, 0) x (1, 0, 0)
  line L0 (913, -137.5) -> (0, -137.5) projected
  circle A0 centre (855.5, -102.75) radius 5.8396
  circle A1 centre (741.5, -102.75) radius 5.8396
  circle A2 centre (627.5, -102.75) radius 5.8396
  circle A3 centre (513.5, -102.75) radius 5.8396
  line L1 (456.5, -137.5) -> (456.5, -188.3524) construction
  circle A4 centre (57.5, -102.75) radius 5.8396
  circle A5 centre (171.5, -102.75) radius 5.8396
  circle A6 centre (285.5, -102.75) radius 5.8396
  circle A7 centre (399.5, -102.75) radius 5.8396
  line L2 (913, 0) -> (913, -137.5) projected
  line L3 (0, 0) -> (913, 0) projected
  point P0 (456.5, 0)
  dimension "d377" = 114
  dimension "d378" = 114
  dimension "d379" = 114
  dimension "d380" = 57
  dimension "d388" = 34.75
  dimension "d389" = 57.5
  dimension "d401" = 102.75
  constraints: 8 centre point, 4 symmetric about line, 3 equal radius, 3 horizontal alignment, 2 end point, 1 midpoint, 1 vertical, 4 other
  measures "d377" distance of A2.centre A3.centre
  measures "d378" distance of A2.centre A1.centre
  measures "d379" distance of A0.centre A1.centre
  measures "d380" distance from line of L1 A3.centre
  measures "d388" distance from line of A0.centre L0
  measures "d389" distance from line of A0.centre L2
  measures "d401" distance from line of L3 A0.centre
hole "Hole15" at (399, 228, 102.75) at (285, 228, 102.75) at (171, 228, 102.75) at (57, 228, 102.75) at (-57, 228, 102.75) at (-171, 228, 102.75) at (-399, 228, 102.75) at (-285, 228, 102.75) direction (0, -1, 0) diameter 10.106 depth 30 tip angle 118 thread size "M12x1.75" class "6H" standard "ISO Metric profile"
chamfer "Chamfer4" distance 2 angle 45 4 edges at (456.5, 228, 68.75) (456.5, -85, 68.75) (-456.5, 228, 68.75) (-456.5, -85, 68.75)
chamfer "Chamfer5" distance 1 angle 45 3 edges at (0, 228, 137.5) (290.25, -85, 137.5) (-290.25, -85, 137.5)
chamfer "Chamfer6" distance 2 angle 45 4 edges at (0, 228, 0) (456.5, 71.5, 0) (0, -85, 0) (-456.5, 71.5, 0)
sketch "Sketch31" plane through (0, 0, 0) normal (0, 0, -1) x (-1, 0, 0)
  circle A0 centre (0, 0) radius 4 projected
  circle A1 centre (-384, 196.75) radius 10 projected
  circle A2 centre (-264, 196.75) radius 10 projected
  line L0 (454.5, 226) -> (454.5, -83) projected
  line L1 (-454.5, -83) -> (-454.5, 226) projected
  line L2 (-454.5, 112) -> (454.5, 112) construction
  circle A3 centre (-324, 196.75) radius 8.0569
  circle A4 centre (-324, 27.25) radius 8.0569
  circle A5 centre (324, 196.75) radius 8.0569
  circle A6 centre (324, 27.25) radius 8.0569
  line L3 (-384, 196.75) -> (-264, 196.75)
  line L4 (-324, 196.75) -> (-324, 110.3967)
  line L5 (-454.5, 71.5) -> (454.5, 71.5)
  circle A7 centre (-144, 196.75) radius 10 projected
  line L6 (-264, 196.75) -> (-144, 196.75)
  line L7 (-204, 196.75) -> (-204, 106.0629)
  circle A8 centre (0, 210) radius 4 projected
  point P0 (0, 0)
  dimension "d408" = 112
  dimension "d410" = 84.75
  dimension "d411" = 324
  dimension "d412" = 84.75
  dimension "d413" = 169.5
  dimension "d421" = 40.5
  dimension "d422" = 204
  dimension "d494" = 324
  dimension "d495" = 196.75
  dimension "d496" = 324
  dimension "d497" = 324
  constraints: 12 end point, 4 centre point, 4 midpoint, 3 equal radius, 3 horizontal, 3 horizontal alignment, 2 point on line, 2 vertical, 2 vertical alignment
  measures "d408" distance from line of L2 A0.centre
  measures "d410" distance from line of L3.start L2
  measures "d411" horizontal distance of A3.centre A0.centre
  measures "d412" distance from line of A4.centre L2
  measures "d413" distance of A4.centre L4.start
  measures "d421" distance between parallel lines of L5 L2
  measures "d422" distance from line of A0.centre L7
  measures "d494" horizontal distance of A5.centre A8.centre
  measures "d495" vertical distance of L4.start A0.centre
  measures "d496" horizontal distance of A4.centre A0.centre
  measures "d497" horizontal distance of A6.centre A0.centre
hole "Hole16" at (324, 196.75, 0) at (324, 27.25, 0) at (-324, 27.25, 0) at (-324, 196.75, 0) direction (0, 0, 1) diameter 10.106 depth 30 tip angle 118 thread size "M12x1.75" class "6H" standard "ISO Metric profile"
chamfer "Chamfer7" distance 1 angle 45 8 edges at (456.5, 29.625, 137.5) (456.5, 214.375, 137.5) (456.5, 155.5, 137.5) (456.5, 179.75, 137.5) (-456.5, 214.375, 137.5) (-456.5, 29.625, 137.5) (-456.5, 179.75, 137.5) (-456.5, 155.5, 137.5)
sketch "Sketch37" plane through (440, 72.475, 127.5) normal (0, 0, 1) x (1, 0, 0)
  circle A0 centre (0, 0) radius 5 projected
  circle A1 centre (0, 0) radius 2
  circle A2 centre (-880, 0) radius 2
  circle A3 centre (-880, 0) radius 5 projected
  point P0 (-440, -72.475)
  dimension "d485" = 4
  dimension "d486" = 4
  constraints: 2 centre point, 1 coincident, 1 concentric
  measures "d485" diameter of A1
  measures "d486" diameter of A2
hole "Hole19" at (440, 72.475, 127.5) at (-440, 72.475, 127.5) direction (0, 0, -1) diameter 3.242 depth 12 tip angle 118 thread size "M4x0.7" class "6H" standard "ANSI Metric M Profile"
body "Solid5"
